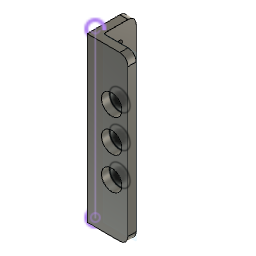
Abstandshalter (Autodesk Fusion 360 design; units mm, degrees)
Autodesk Fusion 360 part; units mm, degrees
sketch "Sketch1" plane through (0, 0, 0) normal (0, 0, 1) x (1, 0, 0)
  line L0 (0, 25) -> (5, 25)
  line L1 (5, 25) -> (5, 5)
  line L2 (5, 0) -> (0, 0)
  line L3 (0, 0) -> (0, 25)
  line L4 (0, 0) -> (25, 0)
  line L5 (25, 0) -> (25, 5)
  line L6 (25, 5) -> (5, 5)
  line L7 (0, 5) -> (0, 0)
  dimension "d1" = 5
  dimension "d6" = 5
  dimension "d7" = 25
  dimension "d8" = 25
  constraint horizontal L0
  constraint vertical L1
  constraint horizontal L2
  constraint vertical L3
  constraint horizontal L4
  constraint vertical L5
  constraint horizontal L6
  constraint vertical L7
  constraint coincident L2.end L3.start
  measures "d1" distance of L0.start L0.end
  measures "d6" distance of L4.end L5.end
  measures "d7" distance of L2.end L0.start
  measures "d8" horizontal distance of L2.end L4.end
extrude "Extrude1" add sketch "Sketch1" along normal blind 100
sketch "Sketch2" plane through (0, 5, 0) normal (0, 1, 0) x (-1, 0, 0)
  line L0 (-25, 0) -> (-5, 0)
  line L1 (-5, 0) -> (-5, 100)
  line L2 (-5, 100) -> (-25, 100)
  line L3 (-25, 100) -> (-25, 0)
  circle A0 centre (-15, 70) radius 6.25
  circle A1 centre (-15, 50) radius 6.25
  circle A2 centre (-15, 30) radius 6.25
  line L4 (0, 0) -> (0, 100)
  dimension "d12" = 12.5
  dimension "d13" = 12.5
  dimension "d14" = 12.5
  dimension "d15" = 20
  dimension "d16" = 20
  dimension "d17" = 30
  dimension "d19" = 10
  dimension "d20" = 10
  dimension "d21" = 10
  dimension "d22" = 30
  dimension "d48" = 15
  measures "d12" diameter of A0
  measures "d13" diameter of A1
  measures "d14" diameter of A2
  measures "d15" vertical distance of A0.centre A1.centre
  measures "d16" distance of A1.centre A2.centre
  measures "d17" distance of L0 A2.centre
  measures "d19" distance of L3 A2.centre
  measures "d20" distance of L3 A1.centre
  measures "d21" distance of L3 A0.centre
  measures "d22" distance of L2 A0.centre
  measures "d48" distance of A1.centre L4
extrude "Extrude2" cut sketch "Sketch2" against normal blind 10 contours A0 | A1 | A2
sketch "Sketch3" plane through (5, 0, 0) normal (1, 0, 0) x (0, 1, 0)
  line L0 (5, 0) -> (25, 0)
  line L1 (25, 0) -> (25, 100)
  line L2 (25, 100) -> (5, 100)
  line L3 (5, 100) -> (5, 0)
  circle A0 centre (15, 10) radius 1.5
  circle A1 centre (15, 50) radius 1.5
  circle A2 centre (15, 90) radius 1.5
  dimension "d25" = 3
  dimension "d26" = 3
  dimension "d27" = 3
  dimension "d28" = 10
  dimension "d29" = 40
  dimension "d30" = 40
  dimension "d32" = 10
  dimension "d33" = 10
  dimension "d34" = 10
  dimension "d35" = 10
  measures "d25" diameter of A0
  measures "d26" diameter of A1
  measures "d27" diameter of A2
  measures "d28" distance of L0 A0.centre
  measures "d29" vertical distance of A0.centre A1.centre
  measures "d30" distance of A1.centre A2.centre
  measures "d32" distance of L1 A2.centre
  measures "d33" distance of L1 A1.centre
  measures "d34" distance of L1 A0.centre
  measures "d35" distance of L2 A2.centre
extrude "Extrude3" cut sketch "Sketch3" against normal blind 10 contours A0 | A1 | A2
fillet "Fillet1" radius 1 1 edges at (5, 5, 50)
fillet "Fillet2" radius 5 1 edges at (2.5, 25, 100)
fillet "Fillet3" radius 5 1 edges at (25, 2.5, 100)
fillet "Fillet4" radius 5 1 edges at (2.5, 25, 0)
fillet "Fillet5" radius 5 1 edges at (25, 2.5, 0)
